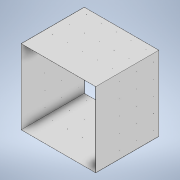
# Autodesk Inventor part: Entrance
Saved by Autodesk Inventor 2022 (Build 260153000, 153)
## iProperties
Created: 2022-03-05
Part Number: Entrance
Material: Generic
Document SubType Name: Modeling
Designer: calvi
Density: 1 g/cm^3
Appearance: Default
Author: calvi
Autodesk Inventor part; units mm, degrees
ref_plane "YZ Plane" through (0, 0, 0) normal (1, 0, 0) x (0, 1, 0)
ref_plane "XZ Plane" through (0, 0, 0) normal (0, 1, 0) x (-1, 0, 0)
ref_plane "XY Plane" through (0, 0, 0) normal (0, 0, 1) x (1, 0, 0)
sketch "Sketch1" plane through (0, 0, 0) normal (0, 0, 1) x (1, 0, 0)
  line L0 (-608.75, -609.5) -> (608.75, 609.5) construction
  line L1 (608.75, -609.5) -> (-608.75, 609.5) construction
  line L2 (-605.75, 606.5) -> (605.75, 606.5)
  line L3 (605.75, 606.5) -> (605.75, -606.5)
  line L4 (605.75, -606.5) -> (-605.75, -606.5)
  line L5 (-605.75, -606.5) -> (-605.75, 606.5)
  point P0 (0, 0)
  dimension "d0" = 1217.5
  dimension "d1" = 1219
  constraints: 12 end point, 2 midpoint, 2 parallel, 1 perpendicular
  measures "d0" distance of L1.end L0.end
  measures "d1" distance of L0.end L1.start
extrude "Extrusion1" add sketch "Sketch1" along normal blind 1025
sketch "Sketch2" plane through (605.75, -606.5, 0) normal (1, 0, 0) x (0, 0, -1)
  line L0 (0, 0) -> (-1025, 0) construction
  line L1 (-639, 0) -> (-639, 1213) construction
  line L2 (0, 1213) -> (-1025, 1213) construction
  line L3 (-364, 0) -> (-364, 1204) construction
  line L4 (-89, 0) -> (-89, 1213) construction
  line L5 (-1025, 0) -> (-1025, 1213) projected
  line L6 (-1025, 122.5) -> (0, 122.5) construction
  line L7 (0, 0) -> (0, 1213) construction
  line L8 (-1025, 364.5) -> (0, 364.5) construction
  line L9 (-1025, 606.5) -> (0, 606.5) construction
  line L10 (-1025, 848.5) -> (0, 848.5) construction
  line L11 (-1025, 1090.5) -> (0, 1090.5) construction
  point P0 (0, 606.5)
  point P1 (-639, 1090.5)
  point P2 (-364, 1090.5)
  point P3 (-89, 1090.5)
  point P4 (-89, 848.5)
  point P5 (-89, 606.5)
  point P6 (-89, 364.5)
  point P7 (-89, 122.5)
  point P8 (-364, 122.5)
  point P9 (-364, 364.5)
  point P10 (-364, 606.5)
  point P11 (-364, 848.5)
  point P12 (-639, 848.5)
  point P13 (-639, 606.5)
  point P14 (-639, 364.5)
  point P15 (-639, 122.5)
  dimension "d5" = 386
  dimension "d6" = 275
  dimension "d7" = 275
  dimension "d8" = 122.5
  dimension "d9" = 242
  dimension "d10" = 242
  dimension "d11" = 242
  dimension "d12" = 242
  dimension "d13" = 122.5
  constraints: 39 point on line, 16 end point, 5 perpendicular, 4 midpoint, 2 vertical, 1 horizontal
  measures "d5" distance between parallel lines of L5 L1
  measures "d6" distance between parallel lines of L3 L1
  measures "d7" distance between parallel lines of L4 L3
  measures "d8" distance between parallel lines of L6 L0
  measures "d9" distance between parallel lines of L8 L6
  measures "d10" distance between parallel lines of L9 L8
  measures "d11" distance between parallel lines of L10 L9
  measures "d12" distance between parallel lines of L11 L10
  measures "d13" distance between parallel lines of L11 L2
sketch "Sketch3" plane through (-605.75, 606.5, 0) normal (0, 1, 0) x (1, 0, 0)
  line L0 (1211.5, -639) -> (0, -639) construction
  line L1 (0, 0) -> (0, -1025) construction
  line L2 (1211.5, -364) -> (7.5, -364) construction
  line L3 (1211.5, -89) -> (0, -89) construction
  line L4 (0, -1025) -> (1211.5, -1025) construction
  line L5 (122.5, -1025) -> (122.5, 0) construction
  line L6 (0, 0) -> (1211.5, 0) construction
  line L7 (364.5, -1000) -> (364.5, 0) construction
  line L8 (606.5, -1000) -> (606.5, 0) construction
  line L9 (848.5, -1025) -> (848.5, 0) construction
  line L10 (1090.5, -1025) -> (1090.5, 0) construction
  line L11 (1211.5, 0) -> (1211.5, -1025) projected
  point P0 (605.75, 0)
  point P1 (122.5, -639)
  point P2 (122.5, -364)
  point P3 (122.5, -89)
  point P4 (364.5, -89)
  point P5 (364.5, -364)
  point P6 (364.5, -639)
  point P7 (606.5, -639)
  point P8 (848.5, -639)
  point P9 (1090.5, -639)
  point P10 (1090.5, -364)
  point P11 (1090.5, -89)
  point P12 (848.5, -89)
  point P13 (848.5, -364)
  point P14 (606.5, -364)
  point P15 (606.5, -89)
  dimension "d14" = 121
  dimension "d15" = 242
  dimension "d16" = 242
  dimension "d17" = 242
  dimension "d18" = 242
  dimension "d19" = 122.5
  constraints: 39 point on line, 16 end point, 3 horizontal, 3 perpendicular, 1 parallel, 1 vertical
  measures "d14" distance between parallel lines of L11 L10
  measures "d15" distance between parallel lines of L10 L9
  measures "d16" distance between parallel lines of L9 L8
  measures "d17" distance between parallel lines of L8 L7
  measures "d18" distance between parallel lines of L7 L5
  measures "d19" distance between parallel lines of L5 L1
shell "Shell1" thickness 1.5 removed faces 2 at (-201.9167, 202.1667, 0) at (-201.9167, 202.1667, 1025)
hole "Hole1" at (605.75, -484, 639) at (605.75, -242, 639) at (605.75, 0, 639) at (605.75, 242, 639) at (605.75, 484, 639) at (605.75, 484, 364) at (605.75, 242, 364) at (605.75, 0, 364) at (605.75, -242, 364) at (605.75, -484, 364) at (605.75, -484, 89) at (605.75, -242, 89) at (605.75, 0, 89) at (605.75, 242, 89) at (605.75, 484, 89) direction (-1, 0, 0) diameter 3 end through all
hole "Hole2" at (-483.25, 606.5, 639) at (-483.25, 606.5, 364) at (-483.25, 606.5, 89) at (-241.25, 606.5, 89) at (-241.25, 606.5, 364) at (-241.25, 606.5, 639) at (0.75, 606.5, 639) at (242.75, 606.5, 639) at (484.75, 606.5, 639) at (484.75, 606.5, 364) at (484.75, 606.5, 89) at (242.75, 606.5, 89) at (242.75, 606.5, 364) at (0.75, 606.5, 364) at (0.75, 606.5, 89) direction (0, -1, 0) diameter 3 end through all
body "Solid1"
